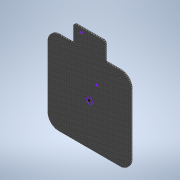
# Autodesk Inventor part: payload_bay_square_drill_holes
Saved by Autodesk Inventor 2020.2 (Build 242310000, 310)
## iProperties
Created: 2020-02-19
Part Number: payload_bay_square_drill_holes
Material: CFRP
Document SubType Name: Modeling
Designer: Krishna Makhija
Density: 1.43 g/cm^3
Appearance: Carbon Fiber
Author: Krishna Makhija
Autodesk Inventor part; units mm, degrees
ref_plane "YZ Plane" through (0, 0, 0) normal (1, 0, 0) x (0, 1, 0)
ref_plane "XZ Plane" through (0, 0, 0) normal (0, 1, 0) x (-1, 0, 0)
ref_plane "XY Plane" through (0, 0, 0) normal (0, 0, 1) x (1, 0, 0)
sketch "Sketch1" plane through (0, 0, 0) normal (0, 0, 1) x (1, 0, 0)
  point P0 (0, 0)
sketch "Sketch2" plane through (0, 0, 0) normal (0, 0, 1) x (1, 0, 0)
  line L0 (94.9998, -95.0001) -> (-94.9998, -95.0001)
  line L1 (-94.9998, -95.0001) -> (-94.9998, 95.0001)
  line L2 (-94.9998, 95.0001) -> (94.9998, 95.0001)
  line L3 (94.9998, 95.0001) -> (94.9998, -95.0001)
  line L4 (94.9998, -95.0001) -> (-94.9998, 95.0001) construction
  line L5 (-94.9998, -95.0001) -> (94.9998, 95.0001) construction
  line L6 (-36.0001, 94.9999) -> (36.0001, 94.9999)
  line L7 (36.0001, 94.9999) -> (36.0001, 135.0001)
  line L8 (36.0001, 135.0001) -> (-36.0001, 135.0001)
  line L9 (-36.0001, 135.0001) -> (-36.0001, 94.9999)
  line L10 (-36.0001, 94.9999) -> (36.0001, 135.0001) construction
  line L11 (36.0001, 94.9999) -> (-36.0001, 135.0001) construction
  point P0 (0, 115)
  point P1 (-36.0001, 95.0001)
  point P2 (36.0001, 95.0001)
  constraints: 24 end point, 4 parallel, 2 horizontal, 2 midpoint, 2 perpendicular
extrude "Extrusion1" add sketch "Sketch2" along normal blind 3
sketch "Standoff holes" plane through (0, 0, 3) normal (0, 0, 1) x (1, 0, 0)
  circle A0 centre (70, 80) radius 1.5001
  circle A1 centre (70, -80) radius 1.5001
  circle A2 centre (-70, 80) radius 1.5001
  circle A3 centre (-70, -80) radius 1.5001
  constraints: 4 centre point
extrude "Extrusion2" cut sketch "Standoff holes" against normal blind 3
fillet "Fillet5" radius 25 4 edges at (-94.9998, 95.0001, 1.5) (94.9998, 95.0001, 1.5) (-94.9998, -95.0001, 1.5) (94.9998, -95.0001, 1.5)
fillet "Fillet6" radius 5 2 edges at (-36.0001, 135.0001, 1.5) (36.0001, 135.0001, 1.5)
sketch "Large Hammond mount holes" plane through (0, 0, 3) normal (0, 0, 1) x (1, 0, 0)
  circle A0 centre (17.6939, 39.717) radius 2.0002
  circle A1 centre (-18.3061, 125.717) radius 2.0002
  constraints: 2 centre point
sketch "BNC flange mount" plane through (0, 0, 3) normal (0, 0, 1) x (1, 0, 0)
  circle A0 centre (0, 0) radius 6.5
  constraints: 1 centre point, 1 coincident
sketch "PX4FLOW mount holes" plane through (0, 0, 0) normal (0, 0, -1) x (-1, 0, 0)
  circle A0 centre (19.5263, 119.2212) radius 1.5872
  circle A1 centre (-4.2863, 119.2212) radius 1.5872
  circle A2 centre (-4.2863, 119.2212) radius 1.5872
  circle A3 centre (-4.2863, 89.0588) radius 1.5872
  circle A4 centre (19.5263, 89.0588) radius 1.5872
  constraints: 5 centre point
sketch "Guard rails mount holes" plane through (0, 0, 0) normal (0, 0, -1) x (-1, 0, 0)
  circle A0 centre (-32.3501, 38.3605) radius 1.2501
  circle A1 centre (-38.3605, 32.3501) radius 1.2501
  circle A2 centre (-60.6344, 66.6448) radius 1.2501
  circle A3 centre (-66.6448, 60.6344) radius 1.2501
  circle A4 centre (-38.3605, -32.3501) radius 1.2501
  circle A5 centre (-32.3501, -38.3605) radius 1.2501
  circle A6 centre (-66.6448, -60.6344) radius 1.2501
  circle A7 centre (-60.6344, -66.6448) radius 1.2501
  circle A8 centre (32.3501, -38.3605) radius 1.2501
  circle A9 centre (38.3605, -32.3501) radius 1.2501
  circle A10 centre (60.6344, -66.6448) radius 1.2501
  circle A11 centre (66.6448, -60.6344) radius 1.2501
  circle A12 centre (38.3605, 32.3501) radius 1.2501
  circle A13 centre (32.3501, 38.3605) radius 1.2501
  circle A14 centre (66.6448, 60.6344) radius 1.2501
  circle A15 centre (60.6344, 66.6448) radius 1.2501
  constraints: 16 centre point
body "Solid1"
